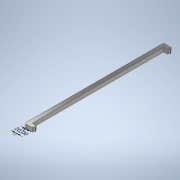
# Autodesk Inventor part: 水平滑台
Saved by Autodesk Inventor 2020 (Build 240168000, 168)
## iProperties
Created: 2021-04-05
Part Number: 水平滑台
Material: 常规
Document SubType Name: Modeling
Designer: 70929
Density: 1 g/cm^3
Appearance: 镀锌
Author: 70929
Autodesk Inventor part; units mm, degrees
ref_plane "YZ Plane" through (0, 0, 0) normal (1, 0, 0) x (0, 1, 0)
ref_plane "XZ Plane" through (0, 0, 0) normal (0, 1, 0) x (-1, 0, 0)
ref_plane "XY Plane" through (0, 0, 0) normal (0, 0, 1) x (1, 0, 0)
sketch "草图1" plane through (0, 0, 0) normal (1, 0, 0) x (0, 1, 0)
  line L0 (-25, 900) -> (25, 900)
  line L1 (25, 900) -> (25, -900)
  line L2 (25, -900) -> (-25, -900)
  line L3 (-25, -900) -> (-25, 900)
  line L4 (-25, 900) -> (25, -900) construction
  line L5 (25, 900) -> (-25, -900) construction
  point P0 (0, 0)
  dimension "d0" = 50
  dimension "d1" = 1800
  constraints: 12 end point, 2 midpoint, 2 parallel, 1 horizontal, 1 perpendicular
  measures "d0" distance of L1.end L2.end
  measures "d1" distance of L0.end L1.end
extrude "拉伸1" add sketch "草图1" against normal mid plane 50
sketch "草图2" plane through (25, 0, 0) normal (1, 0, 0) x (0, 0, -1)
  line L0 (-900, -25) -> (-900, 25) projected
  line L1 (-900, 25) -> (-850, 25)
  line L2 (-850, 25) -> (-850, -25)
  line L3 (-850, -25) -> (-900, -25)
  line L4 (-900, -25) -> (-900, 25)
  line L5 (-900, 25) -> (900, 25) construction
  line L6 (0, 25) -> (0, -25) construction
  line L7 (900, -25) -> (-900, -25) construction
  line L8 (900, -25) -> (900, 25)
  line L9 (900, 25) -> (850, 25)
  line L10 (850, 25) -> (850, -25)
  line L11 (850, -25) -> (900, -25)
  line L12 (900, -25) -> (900, 25)
  line L13 (900, 25) -> (-900, 25) construction
  line L14 (-900, -25) -> (900, -25) construction
  point P0 (0, 0)
  dimension "d4" = 50
  dimension "d5" = 50
  constraints: 24 end point, 7 symmetric about line, 2 midpoint, 2 parallel, 1 horizontal, 1 perpendicular
  measures "d4" distance of L2.end L3.end
  measures "d5" distance of L1.end L2.end
extrude "拉伸2" add sketch "草图2" along normal blind 50
sketch "草图3" plane through (75, 0, 0) normal (1, 0, 0) x (0, 0, -1)
  line L0 (850, 25) -> (850, -25) projected
  line L1 (850, 25) -> (870, 25)
  line L2 (900, 25) -> (880, 25)
  line L3 (870, 25) -> (880, 25)
  line L4 (880, 25) -> (880, -25)
  line L5 (880, -25) -> (870, -25)
  line L6 (870, -25) -> (870, 25)
  line L7 (0, 25) -> (0, -25) construction
  line L8 (-850, 25) -> (-850, -25)
  line L9 (-850, 25) -> (-870, 25)
  line L10 (-900, 25) -> (-880, 25)
  line L11 (-870, 25) -> (-880, 25)
  line L12 (-880, 25) -> (-880, -25)
  line L13 (-880, -25) -> (-870, -25)
  line L14 (-870, -25) -> (-870, 25)
  line L15 (880, -25) -> (870, -25)
  line L16 (850, -25) -> (900, -25) projected
  line L17 (-880, -25) -> (-870, -25)
  line L18 (900, -25) -> (-900, -25) projected
  point P0 (0, 0)
  point P1 (-900, 25)
  point P2 (-850, 25)
  dimension "d10" = 10
  dimension "d11" = 20
  constraints: 32 end point, 8 symmetric about line, 2 horizontal, 2 parallel, 1 collinear, 1 perpendicular, 1 other
  measures "d10" distance between parallel lines of L14 L12
  measures "d11" distance between parallel lines of L8 L14
extrude "拉伸3" add sketch "草图3" along normal blind 15 contours L3 L4 L5 L6 | L14 L13 L12 L11
sketch "草图4" plane through (-25, -25, -900) normal (0, -1, 0) x (1, 0, 0)
  line L0 (0, 0) -> (20, 0)
  line L1 (100, 0) -> (0, 0) projected
  line L2 (20, 0) -> (30, 0)
  line L3 (20, 0) -> (25, 0)
  line L4 (25, 0) -> (25, 1800)
  line L5 (25, 1800) -> (20, 1800)
  line L6 (20, 1800) -> (20, 0)
  line L7 (0, 1800) -> (100, 1800) projected
  point P0 (25, 900)
  dimension "d12" = 20
  dimension "d13" = 10
  dimension "d14" = 5
  dimension "d16" = 1800
  constraints: 12 end point, 2 parallel, 2 point on line, 1 horizontal, 1 perpendicular
  measures "d12" distance of L0.start L0.end
  measures "d13" distance of L0.end L2.end
  measures "d14" distance of L5.end L4.end
  measures "d16" distance between parallel lines of L1 L7
extrude "拉伸4" cut sketch "草图4" against normal blind 5
fillet "圆角1" radius 20 2 edges at (-25, 0, 900) (-25, 0, -900)
